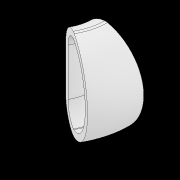
# Autodesk Inventor part: L_Notch-Wedge
Saved by Autodesk Inventor 2021 (Build 250183000, 183)
## iProperties
Created: 2020-11-13
Part Number: L_Notch-Wedge
Material: UHMW, White
Document SubType Name: Modeling
Designer: Eli Mattingly
Density: 0.94 g/cm^3
Appearance: Smooth - White
Author: Eli Mattingly
Autodesk Inventor part; units mm, degrees
ref_plane "Work Plane1" through (-7, 0, -29.5697) normal (1, 0, 0) x (0, 0, -1)
ref_plane "YZ Plane" through (0, 0, 0) normal (1, 0, 0) x (0, 1, 0)
ref_plane "XZ Plane" through (0, 0, 0) normal (0, 1, 0) x (-1, 0, 0)
sketch "Sketch1" plane through (0, 0, 0) normal (0, 0, 1) x (1, 0, 0)
  line L0 (0, 0) -> (0, 22.46) construction
  line L1 (14.7, 11.7) -> (14.7, -11.7)
  line L2 (25.46, 22.46) -> (25.46, -22.46) construction
  arc A0 (24.6721, 22.4311) -> (14.7, 11.7) centre (25.46, 11.7) ccw
  arc A1 (14.7, -11.7) -> (24.6721, -22.4311) centre (25.46, -11.7) ccw
  arc A2 (26.0997, -22.3306) -> (26.0997, 22.3306) centre (21.2486, 0) ccw
  line L3 (0, 0) -> (51.4073, 0)
  arc A3 (26.0997, 22.3306) -> (24.6721, 22.4311) centre (25.0382, 17.4445) ccw
  arc A4 (24.6721, -22.4311) -> (26.0997, -22.3306) centre (25.0382, -17.4445) ccw
  arc A5 (25.4628, 19.399) -> (24.8918, 19.4392) centre (25.0382, 17.4445) ccw
  arc A6 (24.8918, 19.4392) -> (17.7, 11.7) centre (25.46, 11.7) ccw
  line L4 (17.7, 11.7) -> (17.7, -11.7)
  arc A7 (17.7, -11.7) -> (24.8918, -19.4392) centre (25.46, -11.7) ccw
  arc A8 (24.8918, -19.4392) -> (25.4628, -19.399) centre (25.0382, -17.4445) ccw
  arc A9 (25.4628, -19.399) -> (25.4628, 19.399) centre (21.2486, 0) ccw
  point P0 (14.7, 0)
  point P1 (44.1, 0)
  point P2 (25.46, 0)
  dimension "MaxHeight" = 22.46
  dimension "FlatHeightx2" = 23.4
  dimension "ID" = 29.4
  dimension "OD" = 88.2
  dimension "d5" = 44.92
  dimension "RadAtPeak" = 25.46
  dimension "d90" = 5
  dimension "d97" = 3
  constraints: 25 point on circle, 10 centre point, 10 end point, 5 tangent, 3 horizontal alignment, 3 vertical, 2 line through centre, 2 midpoint, 1 equal radius, 1 horizontal, 5 other
  measures "MaxHeight" distance of L0.start L0.end
  measures "FlatHeightx2" distance of L1.start L1.end
  measures "ID" diameter of L1 L0
  measures "OD" diameter of point (44.1, 0) L0
  measures "d5" distance of L2.start L2.end
  measures "RadAtPeak" distance from line of L0.start L2
  measures "d90" radius of A3
  measures "d97" radial gap between concentric circles of A2 A9
revolve "Revolution1" add sketch "Sketch1" angle 30 about axis through (0, 0, 0) along (0, -1, 0) contours A0 A3 A2 L3 A9 A5 A6 L4 L1 | L3 L4 A7 A8 A9 A2 A4 A1 L1
sketch "Sketch13" plane through (14.7, -11.7, 0) normal (0, 0, -1) x (-1, 0, 0)
  arc A0 (0, 23.4) -> (-9.9721, 34.1311) centre (-10.76, 23.4) ccw projected
  arc A1 (-9.9721, 34.1311) -> (-11.3997, 34.0306) centre (-10.3382, 29.1445) ccw projected
  arc A2 (-11.3997, 34.0306) -> (-11.4673, 34.0158) centre (-6.5486, 11.7) ccw projected
  arc A3 (-11.3997, -10.6306) -> (-9.9721, -10.7311) centre (-10.3382, -5.7445) ccw projected
  arc A4 (-9.9721, -10.7311) -> (0, 0) centre (-10.76, 0) ccw projected
  line L0 (0, 23.4) -> (0, 0) projected
  line L1 (-10.76, 0) -> (3, 0)
  line L2 (3, 0) -> (3, 23.4)
  line L3 (3, 23.4) -> (-10.76, 23.4)
  line L4 (-10.76, 23.4) -> (-10.76, 0)
  arc A5 (-11.4673, 34.0158) -> (-11.4673, -10.6158) centre (-6.5486, 11.7) ccw projected
  point P0 (14.7, 11.7)
  point P1 (-7.0149, 11.6038)
  dimension "d93" = 3
  constraints: 8 end point, 2 parallel, 1 horizontal, 1 horizontal alignment, 1 perpendicular, 3 other
  measures "d93" distance between parallel lines of L0 L2
sketch "Sketch7" plane through (0, 0, 0) normal (0, 1, 0) x (-1, 0, 0)
  circle A0 centre (0, 0) radius 198.9616
  constraints: 1 centre point, 1 coincident
sketch "Sketch8" plane through (0, 0, 0) normal (1, 0, 0) x (0, 1, 0)
  circle A0 centre (0, 0) radius 159.0195
  constraints: 1 centre point, 1 coincident
sketch "Sketch9" plane through (0, 0, 0) normal (1, 0, 0) x (0, 0, -1)
  line L0 (74, 0) -> (35, 0) projected
  point P0 (0, 0)
  point P1 (-52.5, 0)
  point P2 (0, 0)
  point P3 (52.5, 0)
  dimension "d88" = 105
  dimension "d89" = 52.5
  constraints: 1 point on line
  measures "d88" distance of point (52.5, 0) point (-52.5, 0)
  measures "d89" distance of point (52.5, 0) point (0, 0)
sketch "Sketch11" plane through (0, 0, 0) normal (1, 0, 0) x (0, 0, -1)
  arc A0 (-35, 25.9107) -> (-42.6927, 34.8921) centre (-44.0893, 25.9107) ccw projected
  line L0 (-35, 25.9107) -> (-35, 0) projected
  line L1 (-35, 0) -> (35, 0) projected
  arc A1 (-50.0415, 0) -> (-54.9585, 0) centre (-52.5, 0) ccw projected
  arc A2 (-50.0415, 0) -> (-54.9585, 0) centre (-37.5, 0) ccw projected
  arc A3 (-39.8678, 39.0634) -> (-73, 0) centre (-33.4058, 0) ccw
  arc A4 (-29.5697, 27.789) -> (-36.4391, 38.3935) centre (-44.0893, 25.9107) ccw
  line L2 (-29.5697, 27.789) -> (-29.5697, 0)
  line L3 (-35, 0) -> (35, 0) projected
  line L4 (-73, 0) -> (-29.5697, 0)
  arc A5 (-36.4391, 38.3935) -> (-39.8678, 39.0634) centre (-39.0518, 34.1304) ccw
  point P0 (0, 0)
  point P1 (-35, 0)
  point P2 (-29.5697, 0)
  point P3 (-54.9585, 0)
  point P4 (-50.0415, 0)
  dimension "d91" = 5
  constraints: 6 point on circle, 4 end point, 3 centre point, 2 tangent, 1 horizontal, 1 point on line, 1 other
  measures "d91" radius of A5
sketch "Sketch6" plane through (5.2886, 0, 3.0534) normal (-0.5, 0, 0.866) x (0, 1, 0)
  line L0 (-11.7, -8.5932) -> (11.7, -8.5932) projected
  arc A0 (-22.3306, -19.9929) -> (22.3306, -19.9929) centre (0, -15.1418) ccw projected
  arc A1 (-23.7082, -22.5925) -> (23.7082, -22.5925) centre (0, -15.1418) ccw
  line L1 (22.3306, -19.9929) -> (21.8002, -19.9929)
  arc A2 (23.7082, -22.5925) -> (21.8002, -19.9929) centre (21.8002, -21.9929) ccw
  line L2 (-21.8002, -19.9929) -> (-22.3306, -19.9929)
  arc A3 (-21.8002, -19.9929) -> (-23.7082, -22.5925) centre (-21.8002, -21.9929) ccw
  line L3 (-34.1227, 6.1068) -> (34.1227, 6.1068) projected
  point P0 (0, 6.1068)
  point P1 (-24.3733, -19.9929)
  point P2 (24.3733, -19.9929)
  point P3 (22.3158, -20.0605)
  point P4 (-22.3158, -20.0605)
  dimension "d47" = 2
  dimension "d48" = 2
  dimension "d49" = 2
  constraints: 8 point on circle, 4 end point, 4 tangent, 3 centre point, 2 point on line, 1 horizontal
  measures "d47" radial gap between concentric circles of A0 A1
  measures "d48" radius of A2
  measures "d49" radius of A3
equation "\"d5\" = 2 * MaxHeight"
equation "\"d63_Copy\" = 35"
body "Solid1"
